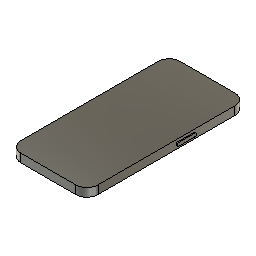
cigarette_case (Autodesk Fusion 360 archive; units mm, degrees)
design "iPhone 14 Pro"
Autodesk Fusion 360 part; units mm, degrees
sketch "Sketch2" plane through (0, 0, 0) normal (0, 0, 1) x (1, 0, 0)
  line L0 (-9.7928, -0.1767) -> (-60.8715, -0.1767)
  line L1 (-71.1163, 10.6723) -> (-71.1163, 137.151)
  line L2 (-60.8715, 148) -> (-9.7928, 148)
  line L3 (0.452, 137.151) -> (0.452, 10.6723)
  line L4 (-71.1163, 73.9117) -> (-45.8836, 73.9117)
  line L5 (-35.3322, -0.1767) -> (-35.3322, 20) construction
  arc A0 (-60.8715, 148) -> (-71.1163, 137.151) centre (-60.8715, 137.7384) ccw
  arc A1 (-71.1163, 10.6723) -> (-60.8715, -0.1767) centre (-60.8715, 10.085) ccw
  arc A2 (0.452, 137.151) -> (-9.7928, 148) centre (-9.7928, 137.7384) ccw
  arc A3 (-9.7928, -0.1767) -> (0.452, 10.6723) centre (-9.7928, 10.085) ccw
  constraint horizontal L0
  constraint vertical L1
  constraint horizontal L2
  constraint vertical L3
  constraint perpendicular L1 L4
  constraint perpendicular L0 L5
  constraint coincident L1 L4.start
  constraint coincident L0 L5.start
  constraint tangent L2 A0
  constraint coincident L2 A0.start
  constraint symmetric L4 L1.end L1.start
  constraint symmetric L4 L2.start L0.end
  constraint symmetric L4 A0 A1
  constraint symmetric L5 L1.end L3.start
  constraint symmetric L5 L2.start L2.end
  constraint symmetric L5 A0 A2
  constraint symmetric L5 L0.end L0.start
  constraint symmetric L5 L1.start L3.end
  constraint symmetric L5 A1 A3
extrude "Extrude2" add sketch "Sketch2" along normal blind 7.85
sketch "Sketch7" plane through (0, 0, 0) normal (0, 0, -1) x (1, 0, 0)
  arc A0 (-60.8715, 0.1767) -> (-71.1163, -10.6723) centre (-60.8715, -10.085) ccw
  line L0 (-71.1163, -10.6723) -> (-71.1163, -137.151)
  arc A1 (-71.1163, -137.151) -> (-60.8715, -148) centre (-60.8715, -137.7384) ccw
  line L1 (-60.8715, -148) -> (-9.7928, -148)
  arc A2 (-9.7928, -148) -> (0.452, -137.151) centre (-9.7928, -137.7384) ccw
  line L2 (0.452, -137.151) -> (0.452, -10.6723)
  arc A3 (0.452, -10.6723) -> (-9.7928, 0.1767) centre (-9.7928, -10.085) ccw
  line L3 (-9.7928, 0.1767) -> (-60.8715, 0.1767)
  arc A4 (-14.3294, -143.9511) -> (-4.3, -135) centre (-14.324, -133.8628) ccw
  line L4 (-14.3294, -143.9511) -> (-32.8176, -143.9412)
  arc A5 (-41.8176, -133.9412) -> (-32.8176, -143.9412) centre (-31.7294, -133.9118) ccw
  arc A6 (-4.1999, -114.9318) -> (-13.1999, -104.9318) centre (-14.2881, -114.9612) ccw
  line L5 (-31.6881, -104.9219) -> (-13.1999, -104.9318)
  arc A7 (-31.6881, -104.9219) -> (-41.7175, -113.873) centre (-31.6935, -115.0101) ccw
  line L6 (-4.3, -135) -> (-4.1999, -114.9318)
  line L7 (-41.8176, -133.9412) -> (-41.7175, -113.873)
  line L8 (-41.7676, -123.9071) -> (-46.5131, -123.9071) construction
  line L9 (-41.7676, -123.9071) -> (-46.5131, -123.9071) construction
  line L10 (0.501, -123.8935) -> (-4.2446, -123.8935) construction
  arc A8 (-3.6999, -114.9323) -> (-13.173, -104.4318) centre (-14.2881, -114.9612) ccw
  line L11 (-31.6878, -104.4219) -> (-13.173, -104.4318)
  arc A9 (-31.6878, -104.4219) -> (-42.2174, -113.8438) centre (-31.6935, -115.0101) ccw
  line L12 (-42.3177, -133.9406) -> (-42.2174, -113.8438)
  arc A10 (-42.3177, -133.9406) -> (-32.8445, -144.4412) centre (-31.7294, -133.9118) ccw
  line L13 (-14.3297, -144.4511) -> (-32.8445, -144.4412)
  arc A11 (-14.3297, -144.4511) -> (-3.8001, -135.0292) centre (-14.324, -133.8628) ccw
  line L14 (-3.8001, -135.0292) -> (-3.6999, -114.9323)
  dimension "d50" = -0.5
  constraint tangent A4 L4
  constraint tangent L5 A7
  constraint parallel L6 L7
  constraint midpoint L7 L8.start
  constraint coincident L6 L10.end
sketch "Sketch4" plane through (-71.1163, 0, 0) normal (-1, 0, 0) x (0, -1, 0)
  line L0 (-137.151, 0) -> (-10.6723, 0)
  line L1 (-10.6723, 7.85) -> (-137.151, 7.85)
  line L2 (-148, 0) -> (-148, 7.85)
  line L3 (-148, 0) -> (-103.41, 0)
  line L4 (-148, 3.925) -> (-89.21, 3.925) construction
  line L5 (-103.41, 0) -> (-103.41, 3.925) construction
  line L6 (-10.6723, 0) -> (-10.6723, 7.85)
  line L7 (-137.151, 7.85) -> (-137.151, 0)
  line L8 (-89.21, 3.925) -> (-89.21, 5.425) construction
  line L9 (-89.21, 3.925) -> (-94.71, 3.925)
  line L10 (-94.71, 3.925) -> (-92.51, 3.925)
  circle A0 centre (-93.61, 3.9249) radius 1.1
  line L11 (-93.61, 5.0249) -> (-89.21, 5.0249)
  line L12 (-93.61, 2.8249) -> (-89.2, 2.8249)
  line L13 (-84.81, 2.8249) -> (-89.22, 2.8249)
  circle A1 centre (-84.81, 3.9249) radius 1.1
  line L14 (-84.81, 5.0249) -> (-89.21, 5.0249)
  line L15 (-89.21, 5.0604) -> (-103.485, 5.0604) construction
  line L16 (-96.3475, 5.0604) -> (-96.3475, 9.5118) construction
  line L17 (-99.085, 5.0249) -> (-103.485, 5.0249)
  circle A2 centre (-99.085, 3.9249) radius 1.1
  line L18 (-99.085, 2.8249) -> (-103.495, 2.8249)
  line L19 (-107.885, 5.0249) -> (-103.485, 5.0249)
  line L20 (-107.885, 2.8249) -> (-103.475, 2.8249)
  circle A3 centre (-107.885, 3.9249) radius 1.1
  line L21 (-120.2472, 3.925) -> (-114, 3.925)
  line L22 (-120.2472, 3.925) -> (-117.1236, 3.925)
  line L23 (-117.1236, 3.925) -> (-117.1236, 5.025)
  line L24 (-117.1236, 5.025) -> (-120.2472, 5.025)
  line L25 (-120.2472, 5.025) -> (-120.2472, 3.925)
  line L26 (-117.1236, 5.025) -> (-114, 5.025)
  line L27 (-114, 5.025) -> (-114, 3.925)
  line L28 (-117.1236, 2.825) -> (-120.2472, 2.825)
  line L29 (-120.2472, 2.825) -> (-120.2472, 3.925)
  line L30 (-117.1236, 2.825) -> (-114, 2.825)
  line L31 (-114, 2.825) -> (-114, 3.925)
  point P0 (-148, 0)
  point P1 (-148, 7.85)
  point P2 (-83.71, 3.925)
  dimension "d32" = 44.59
  dimension "d33" = 58.79
  dimension "d54" = 1.5
  dimension "d55" = 5.5
  dimension "d56" = 2.2
  dimension "d59" = 1.1
  constraint perpendicular L2 L3
  constraint perpendicular L2 L4
  constraint coincident P1 L2.end
  constraint coincident P0 L2.start
  constraint coincident L2 L4.start
  constraint coincident L4 L5.end
  constraint perpendicular L4 L5
  constraint midpoint L2 L4.start
  constraint perpendicular L4 L8
  constraint perpendicular L8 L9
  constraint parallel L9 L10
  constraint coincident L10.end A0
  constraint coincident L9.end A0
  constraint coincident A0 L11.start
  constraint coincident L8 L11.end
  constraint tangent A0 L11
  constraint perpendicular L8 L11
  constraint coincident A0 L12.start
  constraint tangent A0 L12
  constraint parallel L9 L12
  constraint symmetric L8 L9.end P2
  constraint symmetric L8 A0 A1
  constraint symmetric L8 L11.start L14.start
  constraint symmetric L8 L11.end L14.end
  constraint symmetric L8 L12.start L13.start
  constraint symmetric L8 L12.end L13.end
  constraint coincident L8 L15.start
  constraint perpendicular L5 L15
  constraint midpoint L15 L16.start
  constraint perpendicular L15 L16
  constraint symmetric A0 L16 A2
  constraint symmetric L11.start L16 L17.start
  constraint symmetric L11.end L16 L17.end
  constraint symmetric L12.start L16 L18.start
  constraint symmetric L12.end L16 L18.end
  constraint symmetric L13.start L16 L20.start
  constraint symmetric L13.end L16 L20.end
  constraint symmetric A1 L16 A3
  constraint symmetric L14.start L16 L19.start
  constraint coincident L4 L21.start
  constraint coincident L4 L21.end
  constraint horizontal L22
  constraint vertical L23
  constraint horizontal L24
  constraint vertical L25
  constraint symmetric L21.start L21.end L23
  constraint symmetric L24.start L23 L26.start
  constraint symmetric L24.end L23 L26.end
  constraint symmetric L22.start L21 L25.end
  constraint symmetric L21 L23.end L28.start
  constraint symmetric L21 L24.end L28.end
  constraint symmetric L21 L26.end L30.end
  constraint coincident L24 L23.end
  measures "d32" distance of P0 L3.end
  measures "d33" distance of L4.start L4.end
  measures "d54" distance of L4.end L8.end
  measures "d55" distance of L4.end L9.end
  measures "d56" distance of L9.end L10.end
  measures "d59" distance of L22.end L23.end
extrude "Extrude4" add sketch "Sketch4" along normal blind 1 contours L9 L10 A0 | L9 L10 A0 | A0 L11 L12 L13 A1 L14 | A1 | L17 A2 L18 L19 L20 A3 | A2 | A3
sketch "Sketch5" plane through (0.452, 0, 0) normal (1, 0, 0) x (0, 1, 0)
  line L0 (10.6723, 0) -> (137.151, 0)
  line L1 (137.151, 7.85) -> (10.6723, 7.85)
  line L2 (147.46, 3.925) -> (91.92, 3.925) construction
  line L3 (91.92, 0) -> (91.92, 7.85) construction
  line L4 (91.92, 3.925) -> (100.92, 3.925) construction
  line L5 (99.42, 5.425) -> (91.92, 5.425)
  line L6 (91.92, 5.425) -> (91.92, 3.925) construction
  line L7 (99.42, 2.425) -> (91.92, 2.425)
  line L8 (84.42, 5.425) -> (91.92, 5.425)
  line L9 (84.42, 2.425) -> (91.92, 2.425)
  arc A0 (99.42, 2.425) -> (99.42, 5.425) centre (99.42, 3.925) ccw
  arc A1 (84.42, 5.425) -> (84.42, 2.425) centre (84.42, 3.925) ccw
  line L10 (137.151, 0) -> (137.151, 7.85)
  line L11 (10.6723, 7.85) -> (10.6723, 0)
  point P0 (148, 7.85)
  point P1 (148, 0)
  dimension "d43" = 55.54
  dimension "d45" = 9
  dimension "d46" = 1.5
  constraint coincident L0 L3.start
  constraint coincident L1 L3.end
  constraint perpendicular L1 L3
  constraint coincident L2.end L3
  constraint horizontal L4
  constraint horizontal L5
  constraint vertical L6
  constraint symmetric L5.end L4 L7.end
  constraint symmetric L5.end L6 L8.end
  constraint symmetric L6 L7.end L9.end
  constraint tangent L7 A0
  constraint symmetric L3 A0 A1
  measures "d43" distance of L2.start L2.end
  measures "d45" distance of L2.end L4.end
  measures "d46" distance of L2.end L5.end
extrude "Extrude6" add sketch "Sketch5" along normal blind 1 contours L5 L7 L8 L9 A0 A1
sketch "Sketch8" plane through (0, -0.1767, 0) normal (0, -1, 0) x (1, 0, 0)
  line L0 (-60.8715, 0) -> (-9.7928, 0)
  line L1 (-9.7928, 0) -> (-9.7928, 7.85)
  line L2 (-9.7928, 7.85) -> (-60.8715, 7.85)
  line L3 (-60.8715, 7.85) -> (-60.8715, 0)
  line L4 (-60.8715, 3.925) -> (-9.7928, 3.925) construction
  line L5 (-35.3322, 7.85) -> (-35.3322, 0) construction
  line L6 (-35.3322, 3.925) -> (-30, 3.925) construction
  line L7 (-30, 3.925) -> (-30, 3.9204)
  line L8 (-32.6605, 2) -> (-35.3322, 2)
  line L9 (-35.3322, 2) -> (-35.3322, 3.925) construction
  line L10 (-32.6605, 5.85) -> (-35.3322, 5.85)
  line L11 (-30, 3.925) -> (-30, 3.9296)
  line L12 (-38.0038, 5.85) -> (-35.3322, 5.85)
  line L13 (-40.6643, 3.925) -> (-40.6643, 3.9296)
  line L14 (-40.6643, 3.925) -> (-40.6643, 3.9204)
  line L15 (-38.0038, 2) -> (-35.3322, 2)
  spline S0 degree 2 poles (-30, 3.925) (-30, 5.85) (-32.6661, 5.85) knots 0 0 0 0.406223 0.406223 0.406223 weights 1 3 1
  spline S1 degree 2 poles (-40.6643, 3.925) (-40.6643, 5.85) (-37.9983, 5.85) knots 0 0 0 0.406223 0.406223 0.406223 weights 1 3 1
  spline S2 degree 2 poles (-40.6643, 3.925) (-40.6643, 2) (-37.9983, 2) knots 0 0 0 0.406223 0.406223 0.406223 weights 1 3 1
  spline S3 degree 2 poles (-30, 3.925) (-30, 2) (-32.6661, 2) knots 0 0 0 0.406223 0.406223 0.406223 weights 1 3 1
  spline S4 degree 2 poles (-27.6643, 3.925) (-27.6643, 5.85) (-24.9983, 5.85) knots 0 0 0 0.406223 0.406223 0.406223 weights 1 3 1
  line L16 (-25.0038, 5.85) -> (-22.3322, 5.85)
  line L17 (-17.6855, 5.8204) -> (-22.3322, 5.85)
  spline S5 degree 2 poles (-15.0194, 3.8954) (-15.0194, 5.8204) (-17.6855, 5.8204) knots 0 0 0 0.406223 0.406223 0.406223 weights 1 3 1
  line L18 (-15.7826, 2.0043) -> (-22.3302, 2.0043)
  line L19 (-25.0001, 2) -> (-22.3302, 2.0043)
  spline S6 degree 2 poles (-27.6643, 3.925) (-27.6643, 2) (-24.9983, 2) knots 0 0 0 0.406222 0.406222 0.406222 weights 1 3 1
  spline S7 degree 2 poles (-50.9393, 3.9689) (-50.9393, 5.8939) (-48.2732, 5.8939) knots 0 0 0 0.406223 0.406223 0.406223 weights 1 3 1
  line L20 (-46.6661, 5.8609) -> (-48.2732, 5.8939)
  spline S8 degree 2 poles (-44, 3.925) (-44, 5.85) (-46.6661, 5.8609) knots 0 0 0 0.406457 0.406457 0.406457 weights 1 3 1
  spline S9 degree 2 poles (-44, 3.925) (-44, 2) (-46.6661, 2) knots 0 0 0 0.406223 0.406223 0.406223 weights 1 3 1
  line L21 (-46.6605, 2) -> (-48.2748, 2)
  spline S10 degree 2 poles (-50.9393, 3.9689) (-50.9409, 2) (-48.2748, 2) knots 0 0 0 0.410006 0.410006 0.410006 weights 1 3 1
  spline S11 degree 2 poles (-15.0194, 3.8954) (-15.0194, 2.0371) (-15.7826, 2.0043) knots 0 0 0 0.231212 0.231212 0.231212 weights 1 2.414136 1
  constraint midpoint L3 L4.start
  constraint midpoint L1 L4.end
  constraint midpoint L2 L5.start
  constraint midpoint L0 L5.end
  constraint horizontal L6
  constraint vertical L7
  constraint horizontal L8
  constraint vertical L9
  constraint midpoint L4 L6.start
  constraint symmetric L4 L6.end L7.start
  constraint symmetric L4 L8.end L10.end
  constraint symmetric L5 L6.end L13.start
  constraint symmetric L5 L8.end L9.start
  constraint symmetric L5 L10.end L12.end
  constraint coincident S0 L10.start
  constraint coincident L10 S0.end
  constraint coincident S0 L11.end
  constraint symmetric L5 S0.end S1.end
  constraint symmetric L5 S0 S1
  constraint symmetric L6 L7.start L11.start
  constraint symmetric L6 S0.end S3.end
  constraint symmetric L6 S0 S3
  constraint symmetric L6 L13.start L14.start
  constraint symmetric L6 S1.end S2.end
  constraint symmetric L6 S1 S2
  constraint coincident S1 L12.start
  constraint coincident S1 L13.end
  constraint coincident S2 L14.end
  constraint coincident S2 L15.start
  constraint coincident S3 L8.start
  constraint coincident S3 L7.end
  constraint horizontal L18
  constraint coincident L17.start S5
  constraint coincident S5.end L17
  constraint coincident L16.start S4
  constraint coincident L19.start S6
  constraint horizontal L21
  constraint coincident L20.start S8
  constraint coincident S8.end L20
  constraint coincident L21.start S9
  constraint coincident L18.end L19.end
  constraint coincident S6.end L19
  constraint coincident S4.end L16
  constraint coincident L16.end L17.end
  constraint coincident S7.end L20.end
  constraint coincident L21.end S10.end
  constraint coincident S7.start S10.start
equation "base_len = 71.45 mm"
equation "side_length = 147.46 mm"
equation "width = 7.85 mm"
equation "len_to_center_power_button = 55.54 mm"
equation "len_to_center_vol_up = 44.59 mm"
equation "len_to_center_vol_dn = 58.79 mm"
equation "cameras_width = 36.71 mm"
equation "cameras_height = 38.24 mm"
equation "width_with_cameras = 12.02 mm"
equation "corner_oval_1 = 13 mm"
equation "corner_oval_2 = 16 mm"
equation "d21 = width"
equation "edge_to_cameras_edge = 44.58 mm"
equation "d32 = len_to_center_vol_up"
equation "d33 = len_to_center_vol_dn"
equation "vol_button_height = 11 mm"
equation "vol_button_width = 3 mm"
equation "d43 = len_to_center_power_button"
equation "power_button_height = 18 mm"
equation "d45 = power_button_height / 2"
equation "d46 = vol_button_width / 2"
equation "vol_button_diam = 2.2 mm"
equation "d54 = vol_button_width / 2"
equation "d55 = vol_button_height / 2"
equation "d56 = vol_button_diam"
equation "features_tolerance = 0.2 mm"
equation "d59 = vol_button_diam / 2"
equation "d60 = 0.75"
equation "d61 = d60"
equation "d62 = d61"
equation "d63 = d60"
